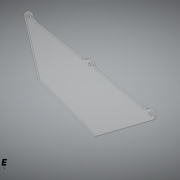
# Autodesk Inventor part: 台形サスカバー
Saved by Autodesk Inventor 2020 (Build 240168000, 168)
## iProperties
Created: 2019-11-14
Part Number: 台形サスカバー
Material: ポリカーボネート、クリア
Document SubType Name: Modeling
Designer: tanjihayato
Density: 1.2 g/cm^3
Appearance: ポリカーボネート - クリア
Mass: 9.40029 g
Surface Area: 109.861 cm^2
Volume: 7.83357 cm^3
Author: tanjihayato
Autodesk Inventor part; units mm, degrees
ref_plane "YZ Plane" through (0, 0, 0) normal (1, 0, 0) x (0, 1, 0)
ref_plane "XZ Plane" through (0, 0, 0) normal (0, 1, 0) x (-1, 0, 0)
ref_plane "XY Plane" through (0, 0, 0) normal (0, 0, 1) x (1, 0, 0)
sketch "スケッチ1" plane through (0, 0, 0) normal (0, 0, 1) x (1, 0, 0)
  circle A0 centre (-35.9404, 22.842) radius 1.5
  circle A1 centre (5.9362, 53.5882) radius 1.5
  circle A2 centre (127.6431, 30.2622) radius 1.5
  line L0 (22.9895, 50.3198) -> (110.5899, 33.5306)
  circle A3 centre (5.9362, 53.5882) radius 4.5
  circle A4 centre (127.6431, 30.2622) radius 4.5
  circle A5 centre (-35.9404, 22.842) radius 3
  line L1 (5.0892, 49.1686) -> (9.9998, 48.2275)
  line L2 (9.9998, 48.2275) -> (22.9895, 50.3198)
  line L3 (110.5899, 33.5306) -> (121.8855, 26.7838)
  line L4 (121.8855, 26.7838) -> (126.7961, 25.8426)
  line L5 (4.4419, 57.8328) -> (15.2047, 61.622)
  line L6 (-37.785, 25.2079) -> (3.1694, 57.1371)
  line L7 (3.5126, 49.7966) -> (-34.0959, 20.4761)
  line L8 (122.0018, 41.1536) -> (130.601, 33.6535)
  circle A6 centre (80.3181, 36.2778) radius 3
  circle A7 centre (80.3181, 36.2778) radius 4.5
  line L9 (128.2106, 34.7263) -> (80.8855, 40.7419)
  circle A8 centre (80.4743, 23.124) radius 1.5
  line L10 (120.4636, 35.711) -> (121.0283, 38.6574)
  line L11 (15.1864, 58.9428) -> (14.6217, 55.9964)
  circle A9 centre (66.9779, 42.9073) radius 1.5
  circle A10 centre (66.9779, 42.9073) radius 3
  line L12 (29.9182, 56.1193) -> (29.3535, 53.1729)
  arc A11 (17.2488, 58.5475) -> (15.1864, 58.9428) centre (16.2176, 58.7451) ccw
  arc A12 (29.9182, 56.1193) -> (27.8558, 56.5146) centre (28.887, 56.3169) ccw
  arc A13 (27.2911, 53.5682) -> (29.3535, 53.1729) centre (28.3223, 53.3705) ccw
  arc A14 (14.6217, 55.9964) -> (16.6841, 55.6011) centre (15.6529, 55.7987) ccw
  line L13 (17.2488, 58.5475) -> (27.8558, 56.5146)
  line L14 (16.6841, 55.6011) -> (27.2911, 53.5682)
  arc A15 (31.8825, 55.7428) -> (27.0019, 58.7146) centre (28.887, 56.3169) ccw
  line L15 (27.0019, 58.7146) -> (18.8556, 60.2759)
  arc A16 (18.8556, 60.2759) -> (15.2047, 61.622) centre (16.2176, 58.7451) ccw
  line L16 (106.2964, 41.4808) -> (105.7317, 38.5345)
  arc A17 (108.3589, 41.0856) -> (106.2964, 41.4808) centre (107.3276, 41.2832) ccw
  arc A18 (121.0283, 38.6574) -> (118.9658, 39.0527) centre (119.997, 38.855) ccw
  arc A19 (118.4011, 36.1063) -> (120.4636, 35.711) centre (119.4323, 35.9086) ccw
  arc A20 (105.7317, 38.5345) -> (107.7942, 38.1392) centre (106.7629, 38.3368) ccw
  line L17 (31.8825, 55.7428) -> (104.3322, 41.8573)
  line L18 (108.3589, 41.0856) -> (118.9658, 39.0527)
  line L19 (107.7942, 38.1392) -> (118.4011, 36.1063)
  arc A21 (122.0018, 41.1536) -> (118.1119, 41.2527) centre (119.997, 38.855) ccw
  line L20 (118.1119, 41.2527) -> (109.9656, 42.814)
  arc A22 (109.9656, 42.814) -> (104.3322, 41.8573) centre (107.3276, 41.2832) ccw
  line L21 (30.451, 58.9354) -> (37.6452, 54.6383)
  line L22 (16.7917, 61.7406) -> (29.4611, 59.3124)
  line L23 (120.5711, 41.8505) -> (107.9017, 44.2787)
  line L24 (106.8426, 44.2944) -> (98.5694, 42.9618)
  point P0 (0, 0)
  point P1 (0, 0)
  dimension "d4" = 9
  dimension "d0" = 9
  dimension "d1" = 9
  dimension "d2" = 6
  dimension "d3" = 6
  dimension "d5" = 47.7059
  dimension "d6" = 47.7059
  dimension "d7" = 3
  dimension "d8" = 3
  dimension "d9" = 8.0769
  dimension "d10" = 8.0769
  dimension "d11" = 3
  dimension "d12" = 6
  dimension "d13" = 61.9691
  dimension "d14" = 61.9691
  dimension "d15" = 15
  dimension "d16" = 2.1
  dimension "d17" = 2
  dimension "d18" = 2
  dimension "d19" = 2
  dimension "d20" = 15
  dimension "d21" = 2.1
  dimension "d22" = 7
  dimension "d23" = 2
  dimension "d24" = 2
  dimension "d25" = 5
  dimension "d26" = 5
  dimension "d27" = 160
  dimension "d28" = 160
  dimension "d29" = 160
  dimension "d30" = 160
  constraints: 50 end point, 39 point on circle, 26 tangent, 22 centre point, 13 point on line, 9 perpendicular, 7 parallel, 6 equal radius, 5 coincident, 2 collinear, 5 other
  measures "d0" diameter of A3
  measures "d1" diameter of A4
  measures "d2" diameter of A5
  measures "d3" diameter of A6
  measures "d5" distance of A8.centre A2.centre
  measures "d6" distance of A2.centre A6.centre
  measures "d7" distance of L10.start L10.end
  measures "d8" distance of L11.start L11.end
  measures "d9" distance from line of A2.centre L10
  measures "d10" distance from line of A1.centre L11
  measures "d11" diameter of A9
  measures "d12" diameter of A10
  measures "d13" distance of A2.centre A9.centre
  measures "d14" distance of A1.centre A9.centre
  measures "d15" distance of L12.start L11.start
  measures "d16" diameter of A11
  measures "d17" distance between parallel lines of L13 L15
  measures "d18" radial gap between concentric circles of A11 A16
  measures "d19" radial gap between concentric circles of A12 A15
  measures "d20" distance of L10.end L16.start
  measures "d21" diameter of A17
  measures "d22" distance between parallel lines of L0 L17
  measures "d23" distance between parallel lines of L18 L20
  measures "d24" radial gap between concentric circles of A21 A18
  measures "d25" distance of L1.start L1.end
  measures "d26" distance of L3.end L4.end
  measures "d27" angle of L4 L3
  measures "d28" angle of L1 L2
  measures "d29" angle of L21 L17
  measures "d30" angle of L17 L24
sketch "スケッチ2" plane through (0, 0, 0) normal (0, 0, 1) x (1, 0, 0)
  circle A0 centre (5.9362, 53.5882) radius 1.5 projected
  circle A1 centre (66.9779, 42.9073) radius 1.5 projected
  circle A2 centre (127.6431, 30.2622) radius 1.5 projected
  arc A3 (10.3689, 52.8126) -> (1.6172, 52.3248) centre (5.9362, 53.5882) ccw
  arc A4 (71.3832, 41.9891) -> (62.5453, 43.6829) centre (66.9779, 42.9073) ccw
  arc A5 (130.338, 26.6583) -> (123.2378, 31.1804) centre (127.6431, 30.2622) ccw
  line L0 (10.3689, 52.8126) -> (62.5453, 43.6829)
  line L1 (71.3832, 41.9891) -> (123.2378, 31.1804)
  line L2 (130.338, 26.6583) -> (72.4655, -16.6159)
  line L3 (72.4655, -16.6159) -> (15.6298, 4.4202)
  line L4 (15.6298, 4.4202) -> (1.6172, 52.3248)
  point P0 (0, 0)
  dimension "d31" = 9
  dimension "d32" = 9
  dimension "d33" = 9
  constraints: 10 end point, 6 point on circle, 4 point on line, 3 centre point, 3 coincident, 2 tangent
  measures "d31" diameter of A3
  measures "d32" diameter of A4
  measures "d33" diameter of A5
extrude "押し出し1" add sketch "スケッチ2" along normal blind 1.5
fillet "フィレット1" radius 5 4 edges at (10.3689, 52.8126, 0.75) (62.5453, 43.6829, 0.75) (71.3832, 41.9891, 0.75) (123.2378, 31.1804, 0.75)
equation "\"d6\" = d5"
equation "\"d10\" = d9"
equation "\"d14\" = d13"
